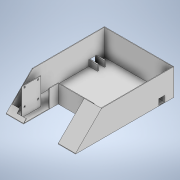
# Autodesk Inventor part: Chasisneww
Saved by Autodesk Inventor 2022 (Build 260153000, 153)
## iProperties
Created: 2021-04-12
Part Number: Chasisneww
Material: Genérico
Document SubType Name: Modeling
Designer: dcast
Density: 1 g/cm^3
Appearance: Valor por defecto
Author: dcast
Autodesk Inventor part; units mm, degrees
ref_plane "YZ Plane" through (0, 0, 0) normal (1, 0, 0) x (0, 1, 0)
ref_plane "XZ Plane" through (0, 0, 0) normal (0, 1, 0) x (-1, 0, 0)
ref_plane "XY Plane" through (0, 0, 0) normal (0, 0, 1) x (1, 0, 0)
sketch "Boceto1" plane through (0, 0, 0) normal (0, 1, 0) x (-1, 0, 0)
  line L0 (-60, 85) -> (-60, -85)
  line L1 (-60, -85) -> (60, -85)
  line L2 (60, -85) -> (60, 85)
  line L3 (-30, 85) -> (-30, 25)
  line L4 (-30, 25) -> (30, 25)
  line L5 (30, 25) -> (30, 85)
  line L6 (60, 85) -> (30, 85)
  line L7 (-30, 85) -> (-60, 85)
  point P0 (0, 0)
  dimension "d0" = 120
  dimension "d1" = 170
  dimension "d2" = 60
  dimension "d4" = 60
  dimension "d5" = 60
  dimension "d6" = 30
  dimension "d11" = 60
  dimension "d12" = 85
  constraints: 16 end point, 5 parallel, 2 horizontal, 2 perpendicular
  measures "d0" distance of L1.end L0.end
  measures "d1" distance of L0.start L0.end
  measures "d2" distance from line of point (0, 0) L2
  measures "d4" distance of L4.end L3.end
  measures "d5" distance of L3.start L3.end
  measures "d6" distance between parallel lines of L2 L5
  measures "d11" distance between parallel lines of L6 L4
  measures "d12" distance from line of point (0, 0) L6
extrude "Extrusión1" add sketch "Boceto1" along normal blind 1
sketch "Boceto2" plane through (0, 1, 0) normal (0, 1, 0) x (1, 0, 0)
  line L0 (-60, 85) -> (-55, 85)
  line L1 (-59, 84) -> (-59, -85)
  line L2 (-59, -85) -> (-60, -85)
  line L3 (-60, -85) -> (-60, 85)
  line L4 (60, -85) -> (60, 85) projected
  line L5 (-60, 85) -> (60, 85)
  line L6 (60, 85) -> (60, 84)
  line L7 (59, 84) -> (-59, 84)
  line L8 (-60, 20) -> (-60, 85)
  line L9 (60, 85) -> (55, 85)
  line L10 (59, 84) -> (59, -85)
  line L11 (59, -85) -> (60, -85)
  line L12 (60, -85) -> (60, 85)
  line L13 (-30, -25) -> (30, -25)
  point P0 (0, 0)
  point P1 (60, -85)
  point P2 (60, 85)
  dimension "d15" = 1
  dimension "d17" = 1
  dimension "d18" = 1
  dimension "d22" = 170
  dimension "d23" = 1
  dimension "d24" = 170
  dimension "d57" = 0
  dimension "d58" = 0
  dimension "d59" = 5
  dimension "d60" = 115
  dimension "d61" = 115
  dimension "d62" = 0
  dimension "d63" = 0
  dimension "d64" = 0
  constraints: 26 end point, 6 parallel, 4 horizontal, 3 perpendicular, 2 point on line
  measures "d15" distance of L1.end L2.end
  measures "d17" distance of L5.end L6.end
  measures "d18" distance of L11.end L10.end
  measures "d22" distance between parallel lines of L9 L11
  measures "d23" distance between parallel lines of L5 L7
  measures "d24" distance between parallel lines of L9 L2
  measures "d57" distance from line of point (60, 85) L4
  measures "d58" distance from line of point (60, -85) L4
  measures "d59" distance from line of L9.end L4
  measures "d60" distance from line of L0.end L4
  measures "d61" distance from line of point (-55, 85) L4
  measures "d62" distance from line of point (60, 85) L0
  measures "d63" distance from line of point (60, -85) L11
  measures "d64" distance from line of point (-55, 85) L9
extrude "Extrusión2" add sketch "Boceto2" along normal blind 45
sketch "Sketch37" plane through (0, 1, 0) normal (0, 1, 0) x (1, 0, 0)
  line L0 (-30, -25) -> (30, -25)
  line L1 (30, -24) -> (-30, -24)
  line L2 (-31, -25) -> (-31, -40)
  line L3 (-31, -40) -> (-30, -40)
  line L4 (-30, -40) -> (-30, -25)
  line L5 (30, -25) -> (30, -85) projected
  line L6 (31, -25) -> (31, -40)
  line L7 (31, -40) -> (30, -40)
  line L8 (30, -40) -> (30, -25)
  line L9 (-31, -25) -> (-31, -24)
  line L10 (-31, -24) -> (-30, -24)
  line L11 (30, -24) -> (31, -24)
  line L12 (31, -24) -> (31, -25)
  point P0 (0, 0)
  dimension "d127" = 1
  dimension "d129" = 1
  dimension "d130" = 90
  dimension "d131" = 16
  dimension "d132" = 15
  dimension "d133" = 0
  dimension "d134" = 60
  dimension "d135" = 15
  dimension "d136" = 15
  constraints: 24 end point, 6 parallel, 3 perpendicular, 3 point on line, 1 horizontal
  measures "d127" distance of L3.end L2.end
  measures "d129" distance of L6.end L7.end
  measures "d130" angle of L3 L5
  measures "d131" distance between parallel lines of L11 L7
  measures "d132" distance between parallel lines of L0 L7
  measures "d133" distance from line of L1.start L5
  measures "d134" distance from line of L1.end L5
  measures "d135" distance from line of L6.start L7
  measures "d136" distance from line of L2.start L7
extrude "Extrusion26" add sketch "Sketch37" along normal blind 30
sketch "Sketch39" plane through (0, 1, 0) normal (0, 1, 0) x (1, 0, 0)
  line L0 (-51, -45) -> (-40, -45)
  line L1 (-40, -45) -> (-40, -78)
  line L2 (-40, -78) -> (-51, -78)
  line L3 (-51, -78) -> (-51, -45)
  line L4 (-30, -85) -> (-30, -40) projected
  line L5 (-59, -85) -> (-30, -85) projected
  point P0 (0, 0)
  dimension "d139" = 11
  dimension "d140" = 33
  dimension "d141" = 10
  dimension "d142" = 7
  constraints: 8 end point, 2 parallel, 1 horizontal, 1 perpendicular
  measures "d139" distance of L1.end L2.end
  measures "d140" distance of L0.end L1.end
  measures "d141" distance between parallel lines of L4 L1
  measures "d142" distance between parallel lines of L5 L2
extrude "Extrusion27" add sketch "Sketch39" along normal blind 1
sketch "Sketch42" plane through (-59, 1, 85) normal (1, 0, 0) x (0, 0, -1)
  line L0 (0, 45) -> (169, 45) projected
  line L1 (0, 0) -> (45, 0) construction
  line L2 (45, 0) -> (45, 45) construction
  line L3 (45, 45) -> (0, 45) construction
  line L4 (0, 45) -> (0, 0) construction
  line L5 (0, 0) -> (169, 0) projected
  line L6 (169, 0) -> (169, 45) projected
  line L7 (0, 45) -> (169, 45) projected
  line L8 (0, 0) -> (0, 45) projected
  line L9 (0, -1) -> (0, 0) projected
  line L10 (170, -1) -> (0, -1) projected
  line L11 (170, 45) -> (170, -1) projected
  line L12 (169, 45) -> (170, 45) projected
  line L13 (0, 0) -> (45, 45)
  line L14 (0, 45) -> (0, 0)
  line L15 (0, -1) -> (0, 45) projected
  point P0 (85, -1)
  dimension "d159" = 45
  constraints: 12 end point, 2 parallel, 1 collinear, 1 horizontal, 1 perpendicular, 1 point on line
  measures "d159" distance of L3.end L2.end
extrude "Extrusion30" cut sketch "Sketch42" against normal blind 33.25 contours L0 L13 L8
sketch "Sketch43" plane through (-59, 1, -84) normal (1, 0, 0) x (0, 0, -1)
  line L0 (0, 0) -> (-169, 0) projected
  line L1 (-159.5434, 0) -> (-159.5434, 11.2545) construction
  line L2 (-169, 0) -> (-124, 45) projected
  line L3 (-159.5434, 9.4566) -> (-169, 0)
  line L4 (-169, 0) -> (-168, 0)
  line L5 (-168, 0) -> (-159.0434, 8.9566)
  line L6 (-159.0434, 8.9566) -> (-159.5434, 9.4566)
  point P0 (-84, -1)
  dimension "d162" = 1
  constraints: 10 end point, 4 point on line, 1 collinear, 1 parallel, 1 perpendicular, 1 vertical
  measures "d162" distance of L3.end L4.end
extrude "Extrusion31" add sketch "Sketch43" along normal blind 29
sketch "Sketch45" plane through (-30, 0, 85) normal (1, 0, 0) x (0, 0, -1)
  line L0 (9.4566, 10.4566) -> (0, 1) projected
  line L1 (4.7283, 5.7283) -> (9.4566, 10.4566)
  line L2 (9.4566, 10.4566) -> (9.9566, 9.9566) projected
  line L3 (9.4566, 10.4566) -> (9.9566, 9.9566)
  line L4 (9.9566, 9.9566) -> (5.2283, 5.2283)
  line L5 (1, 1) -> (9.9566, 9.9566) projected
  line L6 (4.7283, 5.7283) -> (5.2283, 5.2283)
  point P0 (85, 0)
  constraints: 8 end point, 1 collinear, 1 midpoint, 1 perpendicular, 1 point on line
extrude "Extrusion33" cut sketch "Sketch45" against normal blind 16
sketch "Sketch46" plane through (0, 2, 0) normal (0, 1, 0) x (1, 0, 0)
  line L0 (-40, -78) -> (-40, -45) projected
  line L1 (-40, -45) -> (-41, -45)
  line L2 (-41, -45) -> (-41, -78)
  line L3 (-41, -78) -> (-40, -78)
  line L4 (-40, -78) -> (-40, -45)
  point P0 (0, 0)
  dimension "d169" = 1
  constraints: 8 end point, 2 parallel, 1 horizontal, 1 perpendicular
  measures "d169" distance of L3.end L2.end
extrude "Extrusion34" add sketch "Sketch46" along normal blind 45
sketch "Sketch47" plane through (-40, 1, 78) normal (1, 0, 0) x (0, 0, -1)
  line L0 (5, 43) -> (28, 43) construction
  line L1 (0, 0) -> (0, 46) projected
  line L2 (5, 14) -> (28, 14) construction
  line L3 (0, 46) -> (33, 46) projected
  circle A0 centre (5, 43) radius 1.5
  circle A1 centre (28, 43) radius 1.5
  circle A2 centre (5, 14) radius 1.5
  circle A3 centre (28, 14) radius 1.5
  point P0 (78, -1)
  dimension "d172" = 23
  dimension "d173" = 5
  dimension "d174" = 29
  dimension "d175" = 3
  dimension "d176" = 3
  dimension "d177" = 3
  dimension "d178" = 3
  dimension "d179" = 3
  constraints: 4 centre point, 4 coincident, 4 end point, 2 horizontal
  measures "d172" distance of L0.start L0.end
  measures "d173" distance from line of L1 L0.start
  measures "d174" distance between parallel lines of L2 L0
  measures "d175" distance between parallel lines of L3 L0
  measures "d176" diameter of A0
  measures "d177" diameter of A1
  measures "d178" diameter of A2
  measures "d179" diameter of A3
extrude "Extrusion35" cut sketch "Sketch47" against normal blind 1
sketch "Sketch50" plane through (60, 0, 85) normal (1, 0, 0) x (0, 0, -1)
  line L0 (0, 1) -> (45, 46) projected
  line L1 (0, 1) -> (45, 46)
  line L2 (169, 46) -> (0, 46) projected
  line L3 (45, 46) -> (0, 46)
  line L4 (0, 46) -> (0, 1)
  line L5 (0, 0) -> (0, 46) projected
  point P0 (85, 0)
  constraints: 6 end point, 3 collinear
extrude "Extrusion36" cut sketch "Sketch50" against normal blind 1
sketch "Sketch51" plane through (59, 1, -84) normal (-1, 0, 0) x (0, 0, 1)
  line L0 (124, 45) -> (169, 0) projected
  line L1 (124, 45) -> (169, 0)
  line L2 (169, 0) -> (168, 0)
  line L3 (169, 0) -> (0, 0) projected
  line L4 (168, 0) -> (123.5, 44.5)
  line L5 (0, 45) -> (124, 45) projected
  line L6 (123.5, 44.5) -> (124, 45)
  point P0 (84, -1)
  dimension "d185" = 1
  constraints: 8 end point, 1 collinear, 1 parallel, 1 perpendicular, 1 point on line
  measures "d185" distance of L0.end L2.end
extrude "Extrusion37" add sketch "Sketch51" along normal blind 29
sketch "Sketch52" plane through (-60, 0, -85) normal (-1, 0, 0) x (0, 0, 1)
  line L0 (169, 1) -> (1, 1) projected
  line L1 (16, 1) -> (26, 1)
  line L2 (26, 1) -> (26, 11)
  line L3 (26, 11) -> (16, 11)
  line L4 (16, 11) -> (16, 1)
  line L5 (1, 1) -> (1, 46) projected
  point P0 (85, 0)
  point P1 (26, 1)
  dimension "d188" = 10
  dimension "d189" = 10
  dimension "d190" = 15
  constraints: 8 end point, 2 parallel, 1 horizontal, 1 perpendicular, 1 point on line
  measures "d188" distance of L3.end L2.end
  measures "d189" distance of L2.end L1.end
  measures "d190" distance between parallel lines of L5 L4
extrude "Extrusion38" cut sketch "Sketch52" against normal blind 120
sketch "Sketch53" plane through (0, 1, 0) normal (0, 1, 0) x (1, 0, 0)
  line L0 (-59, 69) -> (-44, 69)
  line L1 (-44, 69) -> (-44, 71)
  line L2 (-44, 71) -> (-59, 71)
  line L3 (-59, 71) -> (-59, 69)
  line L4 (-59, 59) -> (-59, -84) projected
  line L5 (-59, 59) -> (-44, 59)
  line L6 (-44, 59) -> (-44, 57)
  line L7 (-44, 57) -> (-59, 57)
  line L8 (-59, 57) -> (-59, 59)
  line L9 (59, 69) -> (59, 84) projected
  line L10 (59, 69) -> (44, 69)
  line L11 (44, 69) -> (44, 71)
  line L12 (44, 71) -> (59, 71)
  line L13 (59, 71) -> (59, 69)
  line L14 (59, 69) -> (59, 59) projected
  line L15 (59, 59) -> (44, 59)
  line L16 (44, 59) -> (44, 57)
  line L17 (44, 57) -> (59, 57)
  line L18 (59, 57) -> (59, 59)
  point P0 (0, 0)
  dimension "d193" = 15
  dimension "d194" = 2
  dimension "d195" = 15
  dimension "d196" = 2
  dimension "d197" = 15
  constraints: 32 end point, 8 parallel, 4 horizontal, 4 perpendicular, 2 point on line
  measures "d193" distance of L2.end L1.end
  measures "d194" distance of L1.end L0.end
  measures "d195" distance of L6.end L7.end
  measures "d196" distance of L5.end L6.end
  measures "d197" distance of L11.end L12.end
extrude "Extrusion39" add sketch "Sketch53" along normal blind 10
